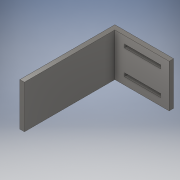
# Autodesk Inventor part: LucasCharles part11 final
Saved by Autodesk Inventor 2018 (Build 220112000, 112)
## iProperties
Created: 2018-05-19
Part Number: LucasCharles part11 final
Material: Stainless Steel, Austenitic
Document SubType Name: Modeling
Designer: Lucas
Density: 8 g/cm^3
Appearance: Semi-Polished
Author: Lucas
Autodesk Inventor part; units mm, degrees
ref_plane "YZ Plane" through (0, 0, 0) normal (1, 0, 0) x (0, 1, 0)
ref_plane "XZ Plane" through (0, 0, 0) normal (0, 1, 0) x (-1, 0, 0)
ref_plane "XY Plane" through (0, 0, 0) normal (0, 0, 1) x (1, 0, 0)
sketch "Sketch1" plane through (0, 0, 0) normal (0, 0, 1) x (1, 0, 0)
  line L0 (0, 0) -> (165.1, 0)
  line L1 (165.1, 0) -> (165.1, 120.65)
  line L2 (165.1, 120.65) -> (0, 120.65)
  line L3 (0, 120.65) -> (0, 0)
  dimension "d0" = 165.1
  dimension "d1" = 120.65
  constraints: 8 end point, 2 parallel, 1 horizontal, 1 perpendicular
  measures "d0" distance of L2.end L1.end
  measures "d1" distance of L1.end L0.end
extrude "Extrusion1" add sketch "Sketch1" against normal blind 12.7
sketch "Sketch2" plane through (0, 0, 0) normal (0, 0, 1) x (1, 0, 0)
  line L0 (165.1, 0) -> (0, 0) projected
  line L1 (0, 120.65) -> (165.1, 120.65) projected
  line L2 (0, 0) -> (12.7, 0)
  line L3 (12.7, 0) -> (12.7, 120.65)
  line L4 (12.7, 120.65) -> (0, 120.65)
  line L5 (0, 120.65) -> (0, 0)
  dimension "d4" = 12.7
  constraints: 8 end point, 2 parallel, 1 horizontal, 1 perpendicular, 1 point on line
  measures "d4" distance of L4.end L3.end
extrude "Extrusion2" add sketch "Sketch2" along normal blind 254
sketch "Sketch5" plane through (0, 0, 0) normal (0, 0, 1) x (1, 0, 0)
  point P0 (0, 0)
sketch "Sketch7" plane through (0, 0, 0) normal (0, 0, 1) x (1, 0, 0)
  line L0 (165.1, 120.65) -> (165.1, 0) projected
  line L1 (165.1, 60.325) -> (0, 60.325)
  line L2 (0, 0) -> (0, 120.65) projected
  line L3 (39.7226, 30.1625) -> (141.3226, 30.1625)
  line L4 (141.3226, 30.1625) -> (141.3226, 20.6375)
  line L5 (141.3226, 20.6375) -> (39.7226, 20.6375)
  line L6 (39.7226, 20.6375) -> (39.7226, 30.1625)
  line L7 (39.7226, 90.4875) -> (141.3226, 90.4875)
  line L8 (141.3226, 90.4875) -> (141.3226, 100.0125)
  line L9 (141.3226, 100.0125) -> (39.7226, 100.0125)
  line L10 (39.7226, 100.0125) -> (39.7226, 90.4875)
  point P0 (118.0813, 25.4)
  point P1 (118.0813, 95.25)
  dimension "d20" = 101.6
  dimension "d21" = 9.525
  dimension "d33" = 4.7625
  dimension "d34" = 4.7625
  constraints: 18 end point, 5 symmetric about line, 2 midpoint, 2 parallel, 1 horizontal, 1 perpendicular
  measures "d20" distance of L4.end L5.end
  measures "d21" distance of L3.end L4.end
  measures "d33" distance from line of L3 point (118.081, 25.4)
  measures "d34" distance from line of L5 point (118.081, 25.4)
hole "Hole1" [suppressed]
extrude "Extrusion7" cut sketch "Sketch7" against normal blind 25.4
sketch "Sketch8" plane through (0, 0, -12.7) normal (-1, 0, 0) x (0, 0, 1)
  line L0 (266.7, 120.65) -> (266.7, 0) projected
  line L1 (266.7, 60.325) -> (0, 60.325)
  line L2 (0, 0) -> (0, 120.65) projected
  line L3 (128.4341, 144.8996) -> (128.4341, -24.2496)
  line L4 (145.5791, 60.325) -> (145.5791, 38.354)
  line L5 (145.5791, 60.325) -> (145.5791, 82.296)
  line L6 (111.2891, 60.325) -> (111.2891, 38.354)
  line L7 (111.2891, 60.325) -> (111.2891, 82.296)
  line L8 (145.5791, 82.296) -> (151.9291, 82.296)
  line L9 (151.9291, 82.296) -> (151.9291, 38.354)
  line L10 (151.9291, 38.354) -> (145.5791, 38.354)
  line L11 (145.5791, 38.354) -> (145.5791, 82.296)
  line L12 (111.2891, 82.296) -> (104.9391, 82.296)
  line L13 (104.9391, 82.296) -> (104.9391, 38.354)
  line L14 (104.9391, 38.354) -> (111.2891, 38.354)
  line L15 (111.2891, 38.354) -> (111.2891, 82.296)
  point P0 (12.7, 0)
  dimension "d35" = 17.145
  dimension "d36" = 21.971
  dimension "d37" = 21.971
  dimension "d38" = 6.35
  dimension "d39" = 6.35
  constraints: 28 end point, 4 parallel, 3 symmetric about line, 3 vertical, 2 horizontal, 2 midpoint, 2 perpendicular, 2 point on line
  measures "d35" distance from line of L3 L4.start
  measures "d36" distance of L4.start L4.end
  measures "d37" distance of L4.start L5.end
  measures "d38" distance of L9.end L10.end
  measures "d39" distance of L14.end L13.end
extrude "Extrusion8" add sketch "Sketch8" along normal blind 38.1
sketch "Sketch9" plane through (0, 38.354, 139.2291) normal (0, 0, 1) x (1, 0, 0)
  line L0 (0, 82.296) -> (0, -38.354) projected
  circle A0 centre (-19.05, 22.7915) radius 6.35
  point P0 (0, 22.7915)
  dimension "d42" = 19.05
  dimension "d43" = 12.7
  constraints: 1 centre point, 1 coincident
  measures "d42" distance from line of L0 point (-19.05, 22.792)
  measures "d43" diameter of A0
extrude "Extrusion9" cut sketch "Sketch9" against normal blind 50.8
body "Solid1"
